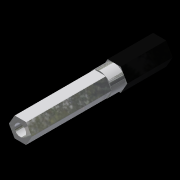
# Autodesk Inventor part: Center Axle
Saved by Autodesk Inventor 2014 SP1 (Build 180222100, 222)
## iProperties
Created: 2013-11-29
Part Number: Center Axle
Material: Aluminum 7075
Document SubType Name: Modeling
Designer: Rauhul Varma
Mass: 18.8317 g
Surface Area: 49.4335 cm^2
Volume: 6.70166 cm^3
Density: 2.81 g/cm^3
Appearance: Aluminum - Polished
Author: Rauhul Varma
Autodesk Inventor part; units mm, degrees
ref_plane "YZ Plane" through (0, 0, 0) normal (1, 0, 0) x (0, 1, 0)
ref_plane "XZ Plane" through (0, 0, 0) normal (0, 1, 0) x (-1, 0, 0)
ref_plane "XY Plane" through (0, 0, 0) normal (0, 0, 1) x (1, 0, 0)
sketch "Sketch1" plane through (0, 0, 0) normal (0, 0, 1) x (1, 0, 0)
  line L0 (-7.3323, 0) -> (-3.6662, 6.35)
  line L1 (-3.6662, 6.35) -> (3.6662, 6.35)
  line L2 (3.6662, 6.35) -> (7.3323, 0)
  line L3 (7.3323, 0) -> (3.6662, -6.35)
  line L4 (3.6662, -6.35) -> (-3.6662, -6.35)
  line L5 (-3.6662, -6.35) -> (-7.3323, 0)
  point P0 (0, 0)
  point P1 (0, 0)
  dimension "d0" = 12.7
  constraints: 12 end point, 1 coincident, 1 horizontal, 13 other
  measures "d0" distance between parallel lines of L4 L1
extrude "Pulley 1/2\" Hex" add sketch "Sketch1" along normal blind 25.4
sketch "Sketch2" plane through (0, 0, 25.4) normal (0, 0, 1) x (1, 0, 0)
  circle A0 centre (0, 0) radius 6.35
  constraints: 1 centre point, 1 coincident
extrude "External 1/2\" Round" add sketch "Sketch2" along normal blind 7.9375
sketch "Sketch3" plane through (0, 0, 33.3375) normal (0, 0, 1) x (1, 0, 0)
  circle A0 centre (0, 0) radius 6.35 projected
  line L0 (3.2748, 5.4404) -> (6.3489, 0.1158)
  line L1 (6.3489, -0.1158) -> (3.2748, -5.4404)
  line L2 (3.0742, -5.5563) -> (-3.0742, -5.5563)
  line L3 (-3.2748, -5.4404) -> (-6.3489, -0.1158)
  line L4 (-6.3489, 0.1158) -> (-3.2748, 5.4404)
  line L5 (-3.0742, 5.5563) -> (3.0742, 5.5563)
  dimension "d5" = 11.1125
  constraints: 12 end point, 1 coincident, 1 horizontal, 20 other
  measures "d5" distance between parallel lines of L2 L5
extrude "Wheel 7/16\" Hex" add sketch "Sketch3" along normal blind 44.45 contours A0 L1 L2 L3 L4 L5 L0
sketch "Sketch4" plane through (0, 0, 77.7875) normal (0, 0, 1) x (1, 0, 0)
  arc A0 (-3.2748, -5.4404) -> (-3.0742, -5.5563) centre (0, 0) ccw projected
  constraints: 1 coincident
hole "Hole1" at (0, 0, 77.7875) direction (0, 0, -1) diameter 6.5278 end through all clearance for "Socket Head Cap Screw" size "1/4" standard "Ansi Unified Screw Threads"
body "Solid1"
